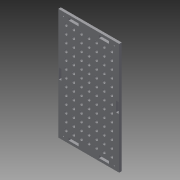
# Autodesk Inventor part: basePanel01
Saved by Autodesk Inventor 2013 (Build 170138000, 138)
## iProperties
Created: 2014-10-07
Part Number: basePanel01
Material: Generic
Document SubType Name: Modeling
Designer: Nano
Density: 1 g/cm^3
Author: Nano
Autodesk Inventor part; units mm, degrees
ref_plane "YZ Plane" through (0, 0, 0) normal (1, 0, 0) x (0, 1, 0)
ref_plane "XZ Plane" through (0, 0, 0) normal (0, 1, 0) x (-1, 0, 0)
ref_plane "XY Plane" through (0, 0, 0) normal (0, 0, 1) x (1, 0, 0)
sketch "Sketch1" plane through (0, 0, 0) normal (0, 0, 1) x (1, 0, 0)
  line L0 (0, -12.7) -> (0, 266.7) projected
  line L1 (-152.4, 266.7) -> (-152.4, -12.7) projected
  line L2 (0, 266.7) -> (-152.4, 266.7) projected
  line L3 (-152.4, -12.7) -> (0, -12.7) projected
  line L4 (-126.6434, 0) -> (-126.6434, -6.35) projected
  line L5 (-126.6434, -6.35) -> (-101.2434, -6.35) projected
  line L6 (-101.2434, -6.35) -> (-101.2434, 0) projected
  line L7 (-101.2434, 0) -> (-126.6434, 0) projected
  line L8 (-50.4434, 0) -> (-50.4434, -6.35) projected
  line L9 (-50.4434, -6.35) -> (-25.0434, -6.35) projected
  line L10 (-25.0434, -6.35) -> (-25.0434, 0) projected
  line L11 (-25.0434, 0) -> (-50.4434, 0) projected
  line L12 (-126.6434, 260.35) -> (-126.6434, 254) projected
  line L13 (-126.6434, 254) -> (-101.2434, 254) projected
  line L14 (-101.2434, 254) -> (-101.2434, 260.35) projected
  line L15 (-101.2434, 260.35) -> (-126.6434, 260.35) projected
  line L16 (-50.4434, 260.35) -> (-50.4434, 254) projected
  line L17 (-50.4434, 254) -> (-25.0434, 254) projected
  line L18 (-25.0434, 254) -> (-25.0434, 260.35) projected
  line L19 (-25.0434, 260.35) -> (-50.4434, 260.35) projected
  circle A0 centre (-12.7, 257.175) radius 1.8542 projected
  circle A1 centre (-139.7, 257.175) radius 1.8542 projected
  circle A2 centre (-139.7, -3.175) radius 1.8542 projected
  circle A3 centre (-12.7, -3.175) radius 1.8542 projected
  point P0 (0, 0)
extrude "Extrusion1" add sketch "Sketch1" along normal blind 6.35
sketch "Sketch2" plane through (0, 0, 6.35) normal (0, 0, 1) x (1, 0, 0)
  line L0 (-150.8125, 139.7) -> (-144.4625, 139.7) projected
  line L1 (-150.8125, 114.3) -> (-150.8125, 139.7) projected
  line L2 (-144.4625, 114.3) -> (-150.8125, 114.3) projected
  line L3 (-144.4625, 139.7) -> (-144.4625, 114.3) projected
  line L4 (-7.9375, 139.7) -> (-1.5875, 139.7) projected
  line L5 (-7.9375, 114.3) -> (-7.9375, 139.7) projected
  line L6 (-1.5875, 114.3) -> (-7.9375, 114.3) projected
  line L7 (-1.5875, 139.7) -> (-1.5875, 114.3) projected
  point P0 (0, 0)
extrude "Extrusion2" cut sketch "Sketch2" against normal through all
sketch "Sketch3" plane through (0, 0, 6.35) normal (0, 0, 1) x (1, 0, 0)
  line L0 (0, -12.7) -> (0, 266.7) projected
  line L1 (0, 266.7) -> (-152.4, 266.7) projected
  line L2 (-152.4, 266.7) -> (-152.4, -12.7) projected
  line L3 (-152.4, -12.7) -> (0, -12.7) projected
  circle A0 centre (-133.35, 241.3) radius 3.9688
  circle A1 centre (-133.35, 222.25) radius 3.9688
  circle A2 centre (-133.35, 203.2) radius 3.9688
  circle A3 centre (-133.35, 184.15) radius 3.9688
  circle A4 centre (-133.35, 165.1) radius 3.9688
  circle A5 centre (-133.35, 146.05) radius 3.9688
  circle A6 centre (-133.35, 127) radius 3.9688
  circle A7 centre (-133.35, 107.95) radius 3.9688
  circle A8 centre (-133.35, 88.9) radius 3.9688
  circle A9 centre (-133.35, 69.85) radius 3.9688
  circle A10 centre (-133.35, 50.8) radius 3.9688
  circle A11 centre (-133.35, 31.75) radius 3.9688
  circle A12 centre (-133.35, 12.7) radius 3.9688
  circle A13 centre (-114.3, 241.3) radius 3.9688
  circle A14 centre (-114.3, 222.25) radius 3.9688
  circle A15 centre (-114.3, 203.2) radius 3.9688
  circle A16 centre (-114.3, 184.15) radius 3.9688
  circle A17 centre (-114.3, 165.1) radius 3.9688
  circle A18 centre (-114.3, 146.05) radius 3.9688
  circle A19 centre (-114.3, 127) radius 3.9688
  circle A20 centre (-114.3, 107.95) radius 3.9688
  circle A21 centre (-114.3, 88.9) radius 3.9688
  circle A22 centre (-114.3, 69.85) radius 3.9688
  circle A23 centre (-114.3, 50.8) radius 3.9688
  circle A24 centre (-114.3, 31.75) radius 3.9688
  circle A25 centre (-114.3, 12.7) radius 3.9688
  circle A26 centre (-95.25, 241.3) radius 3.9688
  circle A27 centre (-95.25, 222.25) radius 3.9688
  circle A28 centre (-95.25, 203.2) radius 3.9688
  circle A29 centre (-95.25, 184.15) radius 3.9688
  circle A30 centre (-95.25, 165.1) radius 3.9688
  circle A31 centre (-95.25, 146.05) radius 3.9688
  circle A32 centre (-95.25, 127) radius 3.9688
  circle A33 centre (-95.25, 107.95) radius 3.9688
  circle A34 centre (-95.25, 88.9) radius 3.9688
  circle A35 centre (-95.25, 69.85) radius 3.9688
  circle A36 centre (-95.25, 50.8) radius 3.9688
  circle A37 centre (-95.25, 31.75) radius 3.9688
  circle A38 centre (-95.25, 12.7) radius 3.9688
  circle A39 centre (-76.2, 241.3) radius 3.9688
  circle A40 centre (-76.2, 222.25) radius 3.9688
  circle A41 centre (-76.2, 203.2) radius 3.9688
  circle A42 centre (-76.2, 184.15) radius 3.9688
  circle A43 centre (-76.2, 165.1) radius 3.9688
  circle A44 centre (-76.2, 146.05) radius 3.9688
  circle A45 centre (-76.2, 127) radius 3.9688
  circle A46 centre (-76.2, 107.95) radius 3.9688
  circle A47 centre (-76.2, 88.9) radius 3.9688
  circle A48 centre (-76.2, 69.85) radius 3.9688
  circle A49 centre (-76.2, 50.8) radius 3.9688
  circle A50 centre (-76.2, 31.75) radius 3.9688
  circle A51 centre (-76.2, 12.7) radius 3.9688
  circle A52 centre (-57.15, 241.3) radius 3.9688
  circle A53 centre (-57.15, 222.25) radius 3.9688
  circle A54 centre (-57.15, 203.2) radius 3.9688
  circle A55 centre (-57.15, 184.15) radius 3.9688
  circle A56 centre (-57.15, 165.1) radius 3.9688
  circle A57 centre (-57.15, 146.05) radius 3.9688
  circle A58 centre (-57.15, 127) radius 3.9688
  circle A59 centre (-57.15, 107.95) radius 3.9688
  circle A60 centre (-57.15, 88.9) radius 3.9688
  circle A61 centre (-57.15, 69.85) radius 3.9688
  circle A62 centre (-57.15, 50.8) radius 3.9688
  circle A63 centre (-57.15, 31.75) radius 3.9688
  circle A64 centre (-57.15, 12.7) radius 3.9688
  circle A65 centre (-38.1, 241.3) radius 3.9688
  circle A66 centre (-38.1, 222.25) radius 3.9688
  circle A67 centre (-38.1, 203.2) radius 3.9688
  circle A68 centre (-38.1, 184.15) radius 3.9688
  circle A69 centre (-38.1, 165.1) radius 3.9688
  circle A70 centre (-38.1, 146.05) radius 3.9688
  circle A71 centre (-38.1, 127) radius 3.9688
  circle A72 centre (-38.1, 107.95) radius 3.9688
  circle A73 centre (-38.1, 88.9) radius 3.9688
  circle A74 centre (-38.1, 69.85) radius 3.9688
  circle A75 centre (-38.1, 50.8) radius 3.9688
  circle A76 centre (-38.1, 31.75) radius 3.9688
  circle A77 centre (-38.1, 12.7) radius 3.9688
  circle A78 centre (-19.05, 241.3) radius 3.9688
  circle A79 centre (-19.05, 222.25) radius 3.9688
  circle A80 centre (-19.05, 203.2) radius 3.9688
  circle A81 centre (-19.05, 184.15) radius 3.9688
  circle A82 centre (-19.05, 165.1) radius 3.9688
  circle A83 centre (-19.05, 146.05) radius 3.9688
  circle A84 centre (-19.05, 127) radius 3.9688
  circle A85 centre (-19.05, 107.95) radius 3.9688
  circle A86 centre (-19.05, 88.9) radius 3.9688
  circle A87 centre (-19.05, 69.85) radius 3.9688
  circle A88 centre (-19.05, 50.8) radius 3.9688
  circle A89 centre (-19.05, 31.75) radius 3.9688
  circle A90 centre (-19.05, 12.7) radius 3.9688
  point P0 (0, 0)
  dimension "d4" = 7.9375
  dimension "d7" = 19.05
  dimension "d10" = 19.05
  dimension "d13" = 25.4
  dimension "d14" = 25.4
  dimension "d15" = 19.05
  dimension "d16" = 19.05
  constraints: 91 centre point, 1 horizontal, 1 vertical, 180 other
  measures "d4" diameter of A0
  measures "d7" distance of A0.centre A1.centre
  measures "d10" distance of A0.centre A13.centre
  measures "d13" distance from line of L1 A0.centre
  measures "d14" distance from line of L3 A12.centre
  measures "d15" distance from line of L2 A0.centre
  measures "d16" distance from line of L0 A78.centre
extrude "Extrusion3" cut sketch "Sketch3" against normal through all contours A0 | A1 | A2 | A3 | A4 | A5 | A6 | A7 | A8 | A9 | A10 | A11 | A12 | A13 | A14 | A15 | A16 | A17 | A18 | A19 | A20 | A21 | A22 | A23 | A24 | A25 | A26 | A27 | A28 | A29 | A30 | A31 | A32 | A33 | A34 | A35 | A36 | A37 | A38 | A39 | A40 | A41 | A42 | A43 | A44 | A45 | A46 | A47 | A48 | A49 | A50 | A51 | A52 | A53 | A54 | A55 | A56 | A57 | A58 | A59 | A60 | A61 | A62 | A63 | A64 | A65 | A66 | A67 | A68 | A69 | A70 | A71 | A72 | A73 | A74 | A75 | A76 | A77 | A78 | A79 | A80 | A81 | A82 | A83 | A84 | A85 | A86 | A87 | A88 | A89 | A90
equation "\"d13\" = d14"
equation "\"d15\" = d16"
body "Solid1"
